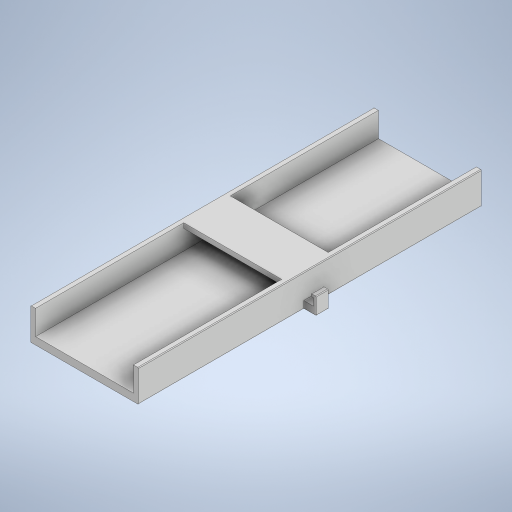
# Autodesk Inventor part: obudowa
Saved by Autodesk Inventor 2024.2 (Build 282272000, 272)
## iProperties
Created: 2024-05-03
Part Number: obudowa
Material: Ogólny
Document SubType Name: Modeling
Designer: kacpe
Density: 1 g/cm^3
Appearance: Domyślna
Author: kacpe
Autodesk Inventor part; units mm, degrees
ref_plane "YZ Plane" through (0, 0, 0) normal (1, 0, 0) x (0, 1, 0)
ref_plane "XZ Plane" through (0, 0, 0) normal (0, 1, 0) x (-1, 0, 0)
ref_plane "XY Plane" through (0, 0, 0) normal (0, 0, 1) x (1, 0, 0)
sketch "Szkic1" plane through (0, 0, 0) normal (0, 1, 0) x (-1, 0, 0)
  line L0 (0, 0) -> (0, -40)
  line L1 (0, 0) -> (44, 0)
  line L2 (44, 0) -> (44, -40)
  line L3 (0, -40) -> (44, -40)
  dimension "d0" = 40
  dimension "d1" = 44
  constraints: 8 end point, 2 vertical, 1 horizontal, 1 perpendicular
  measures "d0" distance of L0.start L0.end
  measures "d1" distance of L0.start L1.end
extrude "Wyciągnięcie proste1" add sketch "Szkic1" along normal blind 3
sketch "Szkic2" plane through (0, 3, 0) normal (0, 1, 0) x (1, 0, 0)
  line L0 (0, 0) -> (0, 40) projected
  line L1 (0, 40) -> (-44, 40) projected
  line L2 (-44, 40) -> (-44, 0) projected
  line L3 (-44, 0) -> (0, 0) projected
  line L4 (-42, 2) -> (-42, 38)
  line L5 (-42, 38) -> (-2, 38)
  line L6 (-2, 38) -> (-2, 2)
  line L7 (-2, 2) -> (-42, 2)
  line L8 (-42, 38) -> (-42, 40)
  line L9 (-2, 38) -> (-2, 40)
  line L10 (-2, 2) -> (-2, 0)
  line L11 (-42, 2) -> (-42, 0)
  dimension "d4" = 2
  constraints: 16 end point, 6 point on line, 1 parallel, 1 vertical, 3 other
  measures "d4" distance between parallel lines of L2 L4
extrude "Wyciągnięcie proste2" add sketch "Szkic2" along normal blind 10 contours L3 L10 L6 L9 L1 L0 | L3 L2 L1 L8 L4 L11
sketch "Szkic3" plane through (0, 0, 0) normal (0, -1, 0) x (1, 0, 0)
  line L0 (0, 0) -> (0, -40) projected
  line L1 (-44, 0) -> (0, 0) projected
  line L2 (-44, -40) -> (-44, 0) projected
  line L3 (0, -40) -> (-44, -40) projected
  line L4 (0, -20) -> (5, -20)
  line L5 (-44, -20) -> (-49, -20) construction
  line L6 (-49, -20) -> (-49, -22.5)
  line L7 (-49, -20) -> (-49, -17.5)
  line L8 (5, -20) -> (5, -22.5)
  line L9 (5, -22.5) -> (5, -20)
  line L10 (5, -20) -> (5, -17.5)
  line L11 (5, -17.5) -> (0, -17.5)
  line L12 (5, -22.5) -> (0, -22.5)
  line L13 (-49, -22.5) -> (-44, -22.5)
  line L14 (-49, -17.5) -> (-44, -17.5)
  dimension "d7" = 5
  dimension "d8" = 5
  dimension "d9" = 2.5
  dimension "d10" = 2.5
  dimension "d11" = 2.5
  dimension "d12" = 2.5
  constraints: 22 end point, 6 point on line, 3 perpendicular, 2 equal length, 2 horizontal, 2 midpoint, 2 vertical
  measures "d7" distance of L4.start L4.end
  measures "d8" distance of L5.start L5.end
  measures "d9" distance of L5.end L6.end
  measures "d10" distance of L5.end L7.end
  measures "d11" distance of L4.end L8.end
  measures "d12" distance of L4.end L10.end
extrude "Wyciągnięcie proste3" add sketch "Szkic3" against normal blind 3 contours L11 L10 L4 L0 | L4 L8 L12 L0 | L2 L13 L6 L7 L14
sketch "Szkic4" plane through (0, 3, 0) normal (0, 1, 0) x (1, 0, 0)
  line L0 (5, 17.5) -> (5, 22.5) projected
  line L1 (5, 22.5) -> (0, 22.5) projected
  line L2 (0, 17.5) -> (0, 22.5) projected
  line L3 (0, 17.5) -> (5, 17.5) projected
  line L4 (5, 17.5) -> (4, 17.5)
  line L5 (4, 17.5) -> (4, 22.5)
  line L6 (4, 22.5) -> (5, 22.5)
  line L7 (5, 22.5) -> (5, 17.5)
  line L8 (-49, 22.5) -> (-49, 17.5) projected
  line L9 (-49, 17.5) -> (-44, 17.5) projected
  line L10 (-44, 22.5) -> (-44, 17.5) projected
  line L11 (-44, 22.5) -> (-49, 22.5) projected
  line L12 (-49, 17.5) -> (-48, 17.5)
  line L13 (-48, 17.5) -> (-48, 22.5)
  line L14 (-48, 22.5) -> (-49, 22.5)
  line L15 (-49, 22.5) -> (-49, 17.5)
  point P0 (0, 0)
  dimension "d15" = 1
  dimension "d16" = 1
  constraints: 16 end point, 4 parallel, 2 horizontal, 2 perpendicular, 2 point on line
  measures "d15" distance of L5.end L6.end
  measures "d16" distance of L14.end L13.end
extrude "Wyciągnięcie proste4" add sketch "Szkic4" along normal blind 4 contours L3 L5 L1 L0 | L11 L13 L9 L8
sketch "Szkic5" plane through (4, 3, -22.5) normal (-1, 0, 0) x (0, 0, 1)
  line L0 (5, 0) -> (0, 0) projected
  line L1 (5, 0) -> (5, 4) projected
  line L2 (0, 4) -> (5, 4) projected
  line L3 (0, 0) -> (0, 4) projected
  line L4 (5, 4) -> (0, 4)
  line L5 (0, 4) -> (0, 3)
  line L6 (0, 3) -> (5, 3)
  line L7 (5, 3) -> (5, 4)
  point P0 (22.5, -3)
  dimension "d19" = 5
  dimension "d20" = 1
  constraints: 8 end point, 2 parallel, 1 horizontal, 1 perpendicular
  measures "d19" distance of L6.end L5.end
  measures "d20" distance of L5.end L4.end
extrude "Wyciągnięcie proste5" add sketch "Szkic5" along normal blind 1 contours L6 L3 L2 L1
sketch "Szkic6" plane through (-48, 3, -17.5) normal (1, 0, 0) x (0, 0, -1)
  line L0 (5, 0) -> (0, 0) projected
  line L1 (5, 0) -> (5, 4) projected
  line L2 (0, 4) -> (5, 4) projected
  line L3 (0, 0) -> (0, 4) projected
  line L4 (0, 4) -> (5, 4)
  line L5 (5, 4) -> (5, 3)
  line L6 (5, 3) -> (0, 3)
  line L7 (0, 3) -> (0, 4)
  point P0 (-17.5, -3)
  point P1 (0, 3)
  point P2 (5, 3)
  dimension "d23" = 5
  dimension "d24" = 1
  constraints: 8 end point, 2 parallel, 1 horizontal, 1 perpendicular
  measures "d23" distance of L5.end L6.end
  measures "d24" distance of L4.end L5.end
extrude "Wyciągnięcie proste6" add sketch "Szkic6" along normal blind 1 contours L6 L3 L2 L1
fillet "Zaokrąglenie1" radius 0.3 18 edges at (-49, 0, -20) (5, 0, -20) (5, 7, -20) (-49, 7, -20) (-44, 0, -31.25) (0, 0, -31.25) (0, 0, -8.75) (2.5, 0, -17.5) (2.5, 0, -22.5) (-44, 0, -8.75) (-46.5, 0, -17.5) (-46.5, 0, -22.5) (0, 13, -20) (-44, 13, -20) (-47, 7, -20) (3, 7, -20) (3, 6, -20) (-47, 6, -20)
sketch "Szkic8" plane through (-42, 3, 0) normal (0, 0, 1) x (1, 0, 0)
  arc A0 (-1.7, 10) -> (-2, 9.7) centre (-1.7, 9.7) ccw projected
  line L0 (-2, -2.7) -> (-2, 9.7) projected
  arc A1 (-2, -2.7) -> (-1.7, -3) centre (-1.7, -2.7) ccw projected
  line L1 (-1.7, -3) -> (41.7, -3) projected
  arc A2 (41.7, -3) -> (42, -2.7) centre (41.7, -2.7) ccw projected
  line L2 (42, -2.7) -> (42, 9.7) projected
  arc A3 (42, 9.7) -> (41.7, 10) centre (41.7, 9.7) ccw projected
  line L3 (40, 10) -> (41.7, 10) projected
  line L4 (40, 0) -> (40, 10) projected
  line L5 (0, 0) -> (40, 0) projected
  line L6 (0, 0) -> (0, 10) projected
  line L7 (-1.7, 10) -> (0, 10) projected
  point P0 (42, -3)
extrude "Wyciągnięcie proste7" add sketch "Szkic8" along normal blind 50
sketch "Szkic9" plane through (-2, 3, -40) normal (0, 0, -1) x (-1, 0, 0)
  arc A0 (42, 9.7) -> (41.7, 10) centre (41.7, 9.7) ccw projected
  line L0 (40, 10) -> (41.7, 10) projected
  line L1 (40, 0) -> (40, 10) projected
  line L2 (0, 0) -> (40, 0) projected
  line L3 (0, 0) -> (0, 10) projected
  line L4 (-1.7, 10) -> (0, 10) projected
  arc A1 (-1.7, 10) -> (-2, 9.7) centre (-1.7, 9.7) ccw projected
  line L5 (-2, -2.7) -> (-2, 9.7) projected
  arc A2 (-2, -2.7) -> (-1.7, -3) centre (-1.7, -2.7) ccw projected
  line L6 (-1.7, -3) -> (41.7, -3) projected
  arc A3 (41.7, -3) -> (42, -2.7) centre (41.7, -2.7) ccw projected
  line L7 (42, -2.7) -> (42, 9.7) projected
  point P0 (-2, -3)
extrude "Wyciągnięcie proste8" add sketch "Szkic9" along normal blind 50
sketch "Szkic10" plane through (0, 13, 0) normal (0, 1, 0) x (1, 0, 0)
  line L0 (-43.7, 90) -> (-43.7, -50) projected
  line L1 (-42, -50) -> (-43.7, -50) projected
  line L2 (-42, 90) -> (-42, -50) projected
  line L3 (-43.7, 90) -> (-42, 90) projected
  line L4 (-2, -50) -> (-2, 90) projected
  line L5 (-2, -50) -> (-2, 90) projected
  line L6 (-42, 90) -> (-2, 90) projected
  line L7 (-42, 90) -> (-42, -50) projected
  line L8 (-2, -50) -> (-42, -50) projected
  line L9 (-44, 22.5) -> (-48, 22.5) projected
  line L10 (-48, 22.5) -> (-48, 17.5) projected
  line L11 (-48, 17.5) -> (-44, 17.5) projected
  line L12 (-44, 22.5) -> (-44, 17.5) projected
  line L13 (-44, 22.5) -> (-48, 22.5) projected
  line L14 (-49, 22.5) -> (-49, 17.5) projected
  line L15 (-48, 22.5) -> (-48, 17.5) projected
  line L16 (-42, 17.5) -> (-2, 17.5)
  line L17 (-2, 17.5) -> (-2, 22.5)
  line L18 (-2, 22.5) -> (-42, 22.5)
  line L19 (-42, 22.5) -> (-42, 17.5)
  line L20 (-42, 17.5) -> (-2, 17.5)
  line L21 (-2, 17.5) -> (-2, 10.5)
  line L22 (-2, 10.5) -> (-42, 10.5)
  line L23 (-42, 10.5) -> (-42, 17.5)
  line L24 (-42, 22.5) -> (-2, 22.5)
  line L25 (-2, 22.5) -> (-2, 29.5)
  line L26 (-2, 29.5) -> (-42, 29.5)
  line L27 (-42, 29.5) -> (-42, 22.5)
  point P0 (0, 0)
  dimension "d32" = 5
  dimension "d33" = 40
  dimension "d34" = 7
  dimension "d35" = 40
  dimension "d36" = 7
  constraints: 24 end point, 6 parallel, 3 horizontal, 3 perpendicular, 2 point on line
  measures "d32" distance of L16.end L17.end
  measures "d33" distance of L21.end L22.end
  measures "d34" distance of L20.end L21.end
  measures "d35" distance of L26.end L25.end
  measures "d36" distance of L25.end L24.end
extrude "Wyciągnięcie proste9" add sketch "Szkic10" against normal blind 2 contours L26 L4 L18 L2 | L2 L16 L4 L22 | L18 L4 L16 L2
